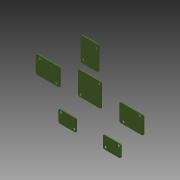
# Autodesk Inventor part: Light Sensors
Saved by Autodesk Inventor 2015 (Build 190159000, 159)
## iProperties
Created: 2016-03-06
Part Number: Light Sensors
Material: Generic
Document SubType Name: Modeling
Designer: James Yelland
Density: 1 g/cm^3
Appearance: Default
Author: James Yelland
Autodesk Inventor part; units mm, degrees
ref_plane "YZ Plane" through (0, 0, 0) normal (1, 0, 0) x (0, 1, 0)
ref_plane "XZ Plane" through (0, 0, 0) normal (0, 1, 0) x (-1, 0, 0)
ref_plane "XY Plane" through (0, 0, 0) normal (0, 0, 1) x (1, 0, 0)
sketch "Sketch1" plane through (0, 0, 0) normal (0, 1, 0) x (-1, 0, 0)
  circle A0 centre (-152.5518, -7.1674) radius 1.6
  circle A1 centre (-131.5518, -24.1674) radius 1.6
  circle A2 centre (-24.5518, -7.1674) radius 1.6
  circle A3 centre (-45.5518, -24.1674) radius 1.6
  circle A4 centre (-97.0518, 40.4352) radius 1.6
  circle A5 centre (-80.0518, 19.4352) radius 1.6
  circle A6 centre (-125.5518, -53.7699) radius 1.6
  circle A7 centre (-108.5518, -63.7699) radius 1.6
  circle A8 centre (-51.5518, -53.7699) radius 1.6
  circle A9 centre (-68.5518, -63.7699) radius 1.6
  line L0 (-155.5518, -4.1674) -> (-128.5518, -4.1674)
  arc A10 (-126.5518, -6.1674) -> (-128.5518, -4.1674) centre (-128.5518, -6.1674) ccw
  line L1 (-126.5518, -6.1674) -> (-126.5518, -25.1674)
  arc A11 (-128.5518, -27.1674) -> (-126.5518, -25.1674) centre (-128.5518, -25.1674) ccw
  line L2 (-128.5518, -27.1674) -> (-155.5518, -27.1674)
  arc A12 (-157.5518, -25.1674) -> (-155.5518, -27.1674) centre (-155.5518, -25.1674) ccw
  line L3 (-157.5518, -25.1674) -> (-157.5518, -6.1674)
  arc A13 (-155.5518, -4.1674) -> (-157.5518, -6.1674) centre (-155.5518, -6.1674) ccw
  line L4 (-21.5518, -4.1674) -> (-48.5518, -4.1674)
  arc A14 (-48.5518, -4.1674) -> (-50.5518, -6.1674) centre (-48.5518, -6.1674) ccw
  line L5 (-50.5518, -6.1674) -> (-50.5518, -25.1674)
  arc A15 (-50.5518, -25.1674) -> (-48.5518, -27.1674) centre (-48.5518, -25.1674) ccw
  line L6 (-48.5518, -27.1674) -> (-21.5518, -27.1674)
  arc A16 (-21.5518, -27.1674) -> (-19.5518, -25.1674) centre (-21.5518, -25.1674) ccw
  line L7 (-19.5518, -25.1674) -> (-19.5518, -6.1674)
  arc A17 (-19.5518, -6.1674) -> (-21.5518, -4.1674) centre (-21.5518, -6.1674) ccw
  line L8 (-77.0518, 16.4352) -> (-77.0518, 43.4352)
  arc A18 (-77.0518, 43.4352) -> (-79.0518, 45.4352) centre (-79.0518, 43.4352) ccw
  line L9 (-79.0518, 45.4352) -> (-98.0518, 45.4352)
  arc A19 (-98.0518, 45.4352) -> (-100.0518, 43.4352) centre (-98.0518, 43.4352) ccw
  line L10 (-100.0518, 43.4352) -> (-100.0518, 16.4352)
  arc A20 (-100.0518, 16.4352) -> (-98.0518, 14.4352) centre (-98.0518, 16.4352) ccw
  line L11 (-98.0518, 14.4352) -> (-79.0518, 14.4352)
  arc A21 (-79.0518, 14.4352) -> (-77.0518, 16.4352) centre (-79.0518, 16.4352) ccw
  line L12 (-126.5518, -50.7699) -> (-107.5518, -50.7699)
  arc A22 (-105.5518, -52.7699) -> (-107.5518, -50.7699) centre (-107.5518, -52.7699) ccw
  line L13 (-105.5518, -52.7699) -> (-105.5518, -64.7699)
  arc A23 (-107.5518, -66.7699) -> (-105.5518, -64.7699) centre (-107.5518, -64.7699) ccw
  line L14 (-107.5518, -66.7699) -> (-126.5518, -66.7699)
  arc A24 (-128.5518, -64.7699) -> (-126.5518, -66.7699) centre (-126.5518, -64.7699) ccw
  line L15 (-128.5518, -64.7699) -> (-128.5518, -52.7699)
  arc A25 (-126.5518, -50.7699) -> (-128.5518, -52.7699) centre (-126.5518, -52.7699) ccw
  line L16 (-50.5518, -50.7699) -> (-69.5518, -50.7699)
  arc A26 (-69.5518, -50.7699) -> (-71.5518, -52.7699) centre (-69.5518, -52.7699) ccw
  line L17 (-71.5518, -52.7699) -> (-71.5518, -64.7699)
  arc A27 (-71.5518, -64.7699) -> (-69.5518, -66.7699) centre (-69.5518, -64.7699) ccw
  line L18 (-69.5518, -66.7699) -> (-50.5518, -66.7699)
  arc A28 (-50.5518, -66.7699) -> (-48.5518, -64.7699) centre (-50.5518, -64.7699) ccw
  line L19 (-48.5518, -64.7699) -> (-48.5518, -52.7699)
  arc A29 (-48.5518, -52.7699) -> (-50.5518, -50.7699) centre (-50.5518, -52.7699) ccw
  line L20 (-88.5518, -24.2699) -> (-101.5518, -24.2699)
  line L21 (-103.5518, -22.2699) -> (-103.5518, 3.7301)
  arc A30 (-103.5518, -22.2699) -> (-101.5518, -24.2699) centre (-101.5518, -22.2699) ccw
  line L22 (-101.5518, 5.7301) -> (-75.5518, 5.7301)
  arc A31 (-101.5518, 5.7301) -> (-103.5518, 3.7301) centre (-101.5518, 3.7301) ccw
  line L23 (-73.5518, 3.7301) -> (-73.5518, -22.2699)
  arc A32 (-75.5518, -24.2699) -> (-73.5518, -22.2699) centre (-75.5518, -22.2699) ccw
  arc A33 (-73.5518, 3.7301) -> (-75.5518, 5.7301) centre (-75.5518, 3.7301) ccw
  line L24 (-75.5518, -24.2699) -> (-88.5518, -24.2699)
  circle A34 centre (-100.5518, 2.7301) radius 1.6
  circle A35 centre (-76.5518, -21.2699) radius 1.6
  constraints: 50 end point, 48 point on circle, 36 centre point
extrude "Extrusion1" add sketch "Sketch1" along normal blind 1
body "Solid1"
